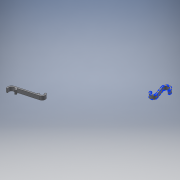
# Autodesk Inventor part: Holders
Saved by Autodesk Inventor 2018 (Build 220112000, 112)
## iProperties
Created: 2018-10-02
Part Number: Holders
Material: Generic
Document SubType Name: Modeling
Designer: eroldan
Density: 1 g/cm^3
Appearance: Default
Author: eroldan
Autodesk Inventor part; units mm, degrees
ref_plane "YZ Plane" through (0, 0, 0) normal (1, 0, 0) x (0, 1, 0)
ref_plane "XZ Plane" through (0, 0, 0) normal (0, 1, 0) x (-1, 0, 0)
ref_plane "XY Plane" through (0, 0, 0) normal (0, 0, 1) x (1, 0, 0)
sketch "Sketch1" plane through (0, 0, 0) normal (0, 0, 1) x (1, 0, 0)
  circle A0 centre (31.9153, 27.3531) radius 7.9375 construction
  circle A1 centre (-47.4702, -19.2083) radius 11.1125 construction
  line L0 (-51.7068, -3.6627) -> (24.1454, 17.0087)
  line L1 (-38.7363, -5.6683) -> (34.3677, 14.6502)
  line L2 (21.6989, 19.4156) -> (24.772, 23.8924)
  line L3 (35.3727, 34.4981) -> (39.058, 38.1402)
  arc A2 (34.3677, 14.6502) -> (39.058, 38.1402) centre (31.9153, 27.3531) ccw
  arc A3 (21.6989, 19.4156) -> (24.1454, 17.0087) centre (31.9153, 27.3531) ccw
  arc A4 (24.772, 23.8924) -> (35.3727, 34.4981) centre (31.9153, 27.3531) ccw
  line L4 (-61.8866, -26.4043) -> (-55.9401, -26.4019)
  line L5 (-32.5458, -13.1359) -> (-36.517, -17.3338)
  arc A5 (-51.7068, -3.6627) -> (-61.8866, -26.4043) centre (-47.4702, -19.2083) ccw
  arc A6 (-32.5458, -13.1359) -> (-38.7363, -5.6683) centre (-47.4702, -19.2083) ccw
  arc A7 (-36.517, -17.3338) -> (-55.9401, -26.4019) centre (-47.4702, -19.2083) ccw
  point P0 (0, 0)
  constraints: 16 point on circle, 12 end point, 6 centre point, 2 concentric, 2 tangent
sketch "Sketch2" plane through (0, 0, 0) normal (0, 0, 1) x (1, 0, 0)
  circle A0 centre (269.3625, 304.1195) radius 11.1125 construction
  circle A1 centre (259.9167, 260.0286) radius 7.9375 construction
  arc A2 (285.4368, 303.0111) -> (254.2353, 298.5715) centre (269.3625, 304.1195) ccw
  arc A3 (247.027, 258.9182) -> (272.0631, 264.4834) centre (259.9167, 260.0286) ccw
  line L0 (258.9295, 300.2932) -> (272.0631, 264.4834)
  line L1 (267.3688, 262.7617) -> (254.2353, 298.5715)
  line L2 (280.0511, 301.0794) -> (285.4368, 303.0111)
  arc A4 (280.0511, 301.0794) -> (258.9295, 300.2932) centre (269.3625, 304.1195) ccw
  line L3 (247.027, 258.9182) -> (252.1016, 261.4168)
  arc A5 (252.1016, 261.4168) -> (267.3688, 262.7617) centre (259.9167, 260.0286) ccw
  dimension "d6" = 5
  dimension "d7" = 5
  constraints: 12 point on circle, 9 end point, 6 centre point, 4 tangent, 1 parallel
  measures "d6" radial gap between concentric circles of A0 A2
  measures "d7" radial gap between concentric circles of A1 A3
extrude "Extrusion2" add sketch "Sketch1" along normal mid plane 15
extrude "Extrusion3" add sketch "Sketch2" along normal mid plane 15 separate body
equation "\"d1\" = d0"
equation "\"d0\" = 5"
